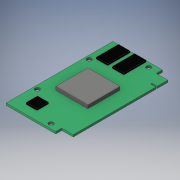
# Autodesk Inventor part: μQ7-962_Module
Saved by Autodesk Inventor 2016 (Build 200138000, 138)
## iProperties
Created: 2017-03-02
Part Number: μQ7-962_Module
Material: Generic
Document SubType Name: Modeling
Designer: jfixelle
Density: 1 g/cm^3
Appearance: Default
Author: jfixelle
Autodesk Inventor part; units mm, degrees
ref_plane "YZ Plane" through (0, 0, 0) normal (1, 0, 0) x (0, 1, 0)
ref_plane "XZ Plane" through (0, 0, 0) normal (0, 1, 0) x (-1, 0, 0)
ref_plane "XY Plane" through (0, 0, 0) normal (0, 0, 1) x (1, 0, 0)
sketch "Sketch1" plane through (0, 0, 0) normal (0, 1, 0) x (-1, 0, 0)
  line L0 (40, 70) -> (0, 70)
  line L1 (0, 70) -> (0, 0)
  line L2 (0, 0) -> (40, 0)
  line L3 (40, 0) -> (40, 70)
  line L4 (0, 4) -> (7.5, 4)
  line L5 (7.5, 4) -> (7.5, 0)
  line L6 (7.5, 0) -> (0, 0)
  line L7 (0, 0) -> (0, 4)
  line L8 (0, 70) -> (7.5, 70)
  line L9 (7.5, 70) -> (7.5, 66)
  line L10 (7.5, 66) -> (0, 66)
  line L11 (0, 66) -> (0, 70)
  line L12 (0, 11) -> (3.0528, 11)
  line L13 (3.5, 11.4472) -> (3.5, 11.8944)
  line L14 (3.0528, 11.8944) -> (0, 11.8944)
  line L15 (0, 11.8944) -> (0, 11)
  arc A0 (3.0528, 11) -> (3.0528, 11.8944) centre (3.0528, 11.4472) ccw
  circle A1 centre (13.5, 3) radius 1.5
  circle A2 centre (13.5, 67) radius 1.5
  circle A3 centre (37.5, 52) radius 1.5
  circle A4 centre (37.5, 18) radius 1.5
  dimension "d0" = 70
  dimension "d1" = 40
  dimension "d2" = 0
  dimension "d3" = 0
  dimension "d4" = 7.5
  dimension "d5" = 7.5
  dimension "d6" = 4
  dimension "d7" = 4
  dimension "d8" = 1
  dimension "d9" = 11
  dimension "d10" = 3.5
  dimension "d13" = 3
  dimension "d14" = 3
  dimension "d15" = 3
  dimension "d16" = 3
  dimension "d17" = 13.5
  dimension "d18" = 13.5
  dimension "d19" = 3
  dimension "d20" = 3
  dimension "d21" = 2.5
  dimension "d22" = 2.5
  dimension "d23" = 18
  dimension "d24" = 18
  constraints: 32 end point, 8 parallel, 5 centre point, 4 horizontal, 4 perpendicular, 3 point on circle, 3 point on line, 3 tangent
  measures "d0" distance of L2.end L0.start
  measures "d1" distance of L1.end L2.end
  measures "d2" distance from line of point (0, 0) L1
  measures "d3" distance from line of point (0, 0) L2
  measures "d4" distance of L9.end L10.end
  measures "d5" distance of L4.start L4.end
  measures "d6" distance of L4.end L5.end
  measures "d7" distance of L8.end L9.end
  measures "d8" distance of L12.end L13.end
  measures "d9" distance between parallel lines of L6 L12
  measures "d10" distance of L13.end L14.end
  measures "d13" distance from line of L2 A1.centre
  measures "d14" distance from line of L0 A2.centre
  measures "d15" diameter of A2
  measures "d16" diameter of A1
  measures "d17" distance from line of L1 A1.centre
  measures "d18" distance from line of L1 A2.centre
  measures "d19" diameter of A3
  measures "d20" diameter of A4
  measures "d21" distance from line of L3 A3.centre
  measures "d22" distance from line of L3 A4.centre
  measures "d23" distance from line of L2 A4.centre
  measures "d24" distance from line of L0 A3.centre
extrude "Extrusion1" add sketch "Sketch1" along normal blind 1.4 contours L3 L2 L5 L4 L1 L12 A0 L14 L10 L9 L0
sketch "Sketch2" plane through (0, 1.4, 0) normal (0, 1, 0) x (1, 0, 0)
  line L0 (-30.8932, -46.4853) -> (-9.8932, -46.4853)
  line L1 (-9.8932, -46.4853) -> (-9.8932, -25.4853)
  line L2 (-9.8932, -25.4853) -> (-30.8932, -25.4853)
  line L3 (-30.8932, -25.4853) -> (-30.8932, -46.4853)
  point P0 (0, 0)
  dimension "d25" = 21
  dimension "d26" = 21
  constraints: 8 end point, 2 parallel, 1 horizontal, 1 perpendicular
  measures "d25" distance of L2.end L0.start
  measures "d26" distance of L1.end L2.end
extrude "Extrusion2" add sketch "Sketch2" along normal blind 2.2
sketch "Sketch3" plane through (0, 1.4, 0) normal (0, 1, 0) x (1, 0, 0)
  line L0 (-35.3745, -15.5245) -> (-27.8702, -15.5245)
  line L1 (-27.8702, -15.5245) -> (-27.8702, -0.887)
  line L2 (-27.8702, -0.887) -> (-35.3745, -0.887)
  line L3 (-35.3745, -0.887) -> (-35.3745, -15.5245)
  line L4 (-24.8422, -15.5245) -> (-17.338, -15.5245)
  line L5 (-17.338, -15.5245) -> (-17.338, -0.887)
  line L6 (-17.338, -0.887) -> (-24.8422, -0.887)
  line L7 (-24.8422, -0.887) -> (-24.8422, -15.5245)
  point P0 (0, 0)
  constraints: 16 end point, 4 parallel, 2 horizontal, 2 perpendicular
extrude "Extrusion3" add sketch "Sketch3" along normal blind 1.1 and the other way blind 2.5
sketch "Sketch4" plane through (0, 1.4, 0) normal (0, 1, 0) x (1, 0, 0)
  line L0 (-32.614, -64.2463) -> (-25.5454, -64.2463)
  line L1 (-25.5454, -64.2463) -> (-25.5454, -56.7849)
  line L2 (-25.5454, -56.7849) -> (-32.614, -56.7849)
  line L3 (-32.614, -56.7849) -> (-32.614, -64.2463)
  point P0 (0, 0)
  constraints: 8 end point, 2 parallel, 1 horizontal, 1 perpendicular
extrude "Extrusion4" add sketch "Sketch4" along normal blind 1.1
sketch "Sketch5" plane through (0, 0, 0) normal (0, -1, 0) x (1, 0, 0)
  line L0 (-38.6782, 35.593) -> (-32.0822, 35.593)
  line L1 (-32.0822, 35.593) -> (-32.0822, 48.5473)
  line L2 (-32.0822, 48.5473) -> (-38.6782, 48.5473)
  line L3 (-38.6782, 48.5473) -> (-38.6782, 35.593)
  point P0 (0, 0)
  constraints: 8 end point, 2 parallel, 1 horizontal, 1 perpendicular
extrude "Extrusion5" add sketch "Sketch5" along normal blind 1.1
body "Solid1"
